Autodesk Inventor part; units mm, degrees
(part 2 of 2)
sketch "Sketch18" plane through (0, 0, -0.2) normal (0, 0, -1) x (-1, 0, 0)
  line L0 (-13.9597, 17.5749) -> (-9.7521, 15.1456) projected
  line L1 (-9.7521, 15.1456) -> (-5.5444, 17.5749) projected
  line L2 (-5.5444, 17.5749) -> (-5.5444, 22.4335) projected
  line L3 (-5.5444, 22.4335) -> (-9.7521, 24.8628) projected
  line L4 (-9.7521, 24.8628) -> (-13.9597, 22.4335) projected
  line L5 (-13.9597, 22.4335) -> (-13.9597, 17.5749) projected
  line L6 (-34.8886, 69.9757) -> (-34.8886, 76.9629) projected
  line L7 (-34.8886, 76.9629) -> (-40.9397, 80.4565) projected
  line L8 (-40.9397, 80.4565) -> (-46.9908, 76.9629) projected
  line L9 (-46.9908, 76.9629) -> (-46.9908, 69.9757) projected
  line L10 (-46.9908, 69.9757) -> (-40.9397, 66.482) projected
  line L11 (-40.9397, 66.482) -> (-34.8886, 69.9757) projected
  line L12 (-49.5403, 66.4665) -> (-49.5403, 71.3251) projected
  line L13 (-49.5403, 71.3251) -> (-53.7479, 73.7544) projected
  line L14 (-53.7479, 73.7544) -> (-57.9556, 71.3251) projected
  line L15 (-57.9556, 71.3251) -> (-57.9556, 66.4665) projected
  line L16 (-57.9556, 66.4665) -> (-53.7479, 64.0372) projected
  line L17 (-53.7479, 64.0372) -> (-49.5403, 66.4665) projected
  line L18 (0, 0) -> (-63.5, 0)
  line L19 (-63.5, 0) -> (-63.5, 88.9)
  line L20 (-63.5, 88.9) -> (0, 88.9)
  line L21 (0, 88.9) -> (0, 0)
  line L22 (-24.4329, 66.1976) -> (-24.4329, 72.4542) projected
  line L23 (-22.5603, 66.482) -> (-16.5092, 69.9757) projected
  line L24 (-16.5092, 69.9757) -> (-16.5092, 76.9629) projected
  line L25 (-16.5092, 76.9629) -> (-22.5603, 80.4565) projected
  line L26 (-22.5603, 80.4565) -> (-28.6114, 76.9629) projected
  line L27 (-28.6114, 76.9629) -> (-28.6114, 69.9757) projected
  line L28 (-28.6114, 69.9757) -> (-22.5603, 66.482) projected
  line L29 (-22.6851, 47.9436) -> (-22.6851, 40.9564) projected
  line L30 (-16.6339, 37.4628) -> (-10.5828, 40.9564) projected
  line L31 (-10.5828, 40.9564) -> (-10.5828, 47.9436) projected
  line L32 (-10.5828, 47.9436) -> (-16.6339, 51.4372) projected
  line L33 (-16.6339, 51.4372) -> (-22.6851, 47.9436) projected
  line L34 (-22.6851, 40.9564) -> (-16.6339, 37.4628) projected
  line L35 (-31.75, 54.2591) -> (-25.6989, 57.7528) projected
  line L36 (-25.6989, 57.7528) -> (-25.6989, 64.74) projected
  line L37 (-25.6989, 64.74) -> (-31.75, 68.2336) projected
  line L38 (-31.75, 68.2336) -> (-37.8011, 64.74) projected
  line L39 (-37.8011, 64.74) -> (-37.8011, 57.7528) projected
  line L40 (-37.8011, 57.7528) -> (-31.75, 54.2591) projected
  spline S0 degree 2 poles (-51.8872, 81.4609) (-51.8872, 81.2551) (-51.9037, 80.9175) (-51.9119, 80.8187) knots 0 0 0 0.5 1 1 1 projected
  spline S1 degree 2 poles (-51.9119, 80.8187) (-52.2906, 80.5635) (-53.2951, 80.2588) (-53.7315, 80.2588) knots 0 0 0 0.5 1 1 1 projected
  spline S2 degree 2 poles (-53.7315, 80.2588) (-54.1102, 80.2588) (-54.7606, 80.3988) (-55.0241, 80.6129) knots 0 0 0 0.5 1 1 1 projected
  spline S3 degree 2 poles (-55.0241, 80.6129) (-55.3864, 80.9093) (-55.7157, 81.7408) (-55.7157, 82.383) knots 0 0 0 0.5 1 1 1 projected
  spline S4 degree 2 poles (-55.7157, 82.383) (-55.7157, 83.5192) (-54.7195, 84.7213) (-53.8797, 84.7213) knots 0 0 0 0.5 1 1 1 projected
  spline S5 degree 2 poles (-53.8797, 84.7213) (-53.5174, 84.7213) (-52.8999, 84.4743) (-52.6035, 84.145) knots 0 0 0 0.5 1 1 1 projected
  spline S6 degree 2 poles (-52.6035, 84.145) (-52.2659, 83.7909) (-51.8872, 82.4901) (-51.8872, 81.4609) knots 0 0 0 0.5 1 1 1 projected
  spline S7 degree 2 poles (-56.1439, 84.8778) (-56.5885, 84.4085) (-57.0989, 83.1076) (-57.0989, 82.3254) knots 0 0 0 0.5 1 1 1 projected
  spline S8 degree 2 poles (-57.0989, 82.3254) (-57.0989, 81.428) (-56.5391, 80.1518) (-55.9957, 79.7319) knots 0 0 0 0.5 1 1 1 projected
  spline S9 degree 2 poles (-55.9957, 79.7319) (-55.5264, 79.3779) (-54.596, 79.1309) (-54.0361, 79.1309) knots 0 0 0 0.5 1 1 1 projected
  spline S10 degree 2 poles (-54.0361, 79.1309) (-53.4515, 79.1309) (-52.4635, 79.4684) (-51.9201, 79.8389) knots 0 0 0 0.5 1 1 1 projected
  spline S11 degree 2 poles (-51.9201, 79.8389) (-52.0272, 78.2087) (-53.5503, 76.4468) (-54.8841, 76.4468) knots 0 0 0 0.5 1 1 1 projected
  spline S12 degree 2 poles (-54.8841, 76.4468) (-55.2546, 76.4468) (-55.9792, 76.6197) (-56.1521, 76.7185) knots 0 0 0 0.5 1 1 1 projected
  line L41 (-56.1521, 76.7185) -> (-56.218, 76.7185) projected
  line L42 (-56.218, 76.7185) -> (-56.218, 75.4094) projected
  spline S13 degree 2 poles (-56.218, 75.4094) (-55.9545, 75.327) (-55.337, 75.2694) (-55.0653, 75.2694) knots 0 0 0 0.5 1 1 1 projected
  spline S14 degree 2 poles (-55.0653, 75.2694) (-53.8632, 75.2694) (-52.2165, 76.101) (-51.632, 76.8914) knots 0 0 0 0.5 1 1 1 projected
  spline S15 degree 2 poles (-51.632, 76.8914) (-51.0803, 77.6406) (-50.5122, 79.8966) (-50.5122, 81.1563) knots 0 0 0 0.5 1 1 1 projected
  spline S16 degree 2 poles (-50.5122, 81.1563) (-50.5122, 82.5477) (-51.0886, 84.3591) (-51.6155, 84.9189) knots 0 0 0 0.5 1 1 1 projected
  spline S17 degree 2 poles (-51.6155, 84.9189) (-52.0354, 85.3635) (-53.1716, 85.8328) (-53.8714, 85.8328) knots 0 0 0 0.5 1 1 1 projected
  spline S18 degree 2 poles (-53.8714, 85.8328) (-54.4972, 85.8328) (-55.724, 85.3306) (-56.1439, 84.8778) knots 0 0 0 0.5 1 1 1 projected
  line L43 (-52.9172, 40.9564) -> (-46.8661, 37.4628) projected
  line L44 (-46.8661, 37.4628) -> (-40.8149, 40.9564) projected
  line L45 (-40.8149, 40.9564) -> (-40.8149, 47.9436) projected
  line L46 (-40.8149, 47.9436) -> (-46.8661, 51.4372) projected
  line L47 (-46.8661, 51.4372) -> (-52.9172, 47.9436) projected
  line L48 (-52.9172, 47.9436) -> (-52.9172, 40.9564) projected
  line L49 (-37.8011, 47.9436) -> (-37.8011, 40.9564) projected
  line L50 (-37.8011, 40.9564) -> (-31.75, 37.4628) projected
  line L51 (-31.75, 37.4628) -> (-25.6989, 40.9564) projected
  line L52 (-25.6989, 40.9564) -> (-25.6989, 47.9436) projected
  line L53 (-25.6989, 47.9436) -> (-31.75, 51.4372) projected
  line L54 (-31.75, 51.4372) -> (-37.8011, 47.9436) projected
  line L55 (-31.75, 34.6409) -> (-37.8011, 31.1472) projected
  line L56 (-37.8011, 31.1472) -> (-37.8011, 24.16) projected
  line L57 (-37.8011, 24.16) -> (-31.75, 20.6664) projected
  line L58 (-31.75, 20.6664) -> (-25.6989, 24.16) projected
  line L59 (-25.6989, 24.16) -> (-25.6989, 31.1472) projected
  line L60 (-25.6989, 31.1472) -> (-31.75, 34.6409) projected
  line L61 (-34.8886, 11.9371) -> (-34.8886, 18.9243) projected
  line L62 (-34.8886, 18.9243) -> (-40.9397, 22.418) projected
  line L63 (-40.9397, 22.418) -> (-46.9908, 18.9243) projected
  line L64 (-46.9908, 18.9243) -> (-46.9908, 11.9371) projected
  line L65 (-46.9908, 11.9371) -> (-40.9397, 8.4435) projected
  line L66 (-40.9397, 8.4435) -> (-34.8886, 11.9371) projected
  line L67 (-28.6114, 11.9371) -> (-22.5603, 8.4435) projected
  line L68 (-22.5603, 8.4435) -> (-16.5092, 11.9371) projected
  line L69 (-16.5092, 11.9371) -> (-16.5092, 18.9243) projected
  line L70 (-16.5092, 18.9243) -> (-22.5603, 22.418) projected
  line L71 (-22.5603, 22.418) -> (-28.6114, 18.9243) projected
  line L72 (-28.6114, 18.9243) -> (-28.6114, 11.9371) projected
  spline S19 degree 2 poles (-11.6128, 7.7837) (-11.6128, 7.9895) (-11.5963, 8.3271) (-11.5881, 8.4259) knots 0 0 0 0.5 1 1 1 projected
  spline S20 degree 2 poles (-11.5881, 8.4259) (-11.2094, 8.6811) (-10.2049, 8.9857) (-9.7685, 8.9857) knots 0 0 0 0.5 1 1 1 projected
  spline S21 degree 2 poles (-9.7685, 8.9857) (-9.3898, 8.9857) (-8.7394, 8.8458) (-8.4759, 8.6317) knots 0 0 0 0.5 1 1 1 projected
  spline S22 degree 2 poles (-8.4759, 8.6317) (-8.1136, 8.3353) (-7.7843, 7.5037) (-7.7843, 6.8615) knots 0 0 0 0.5 1 1 1 projected
  spline S23 degree 2 poles (-7.7843, 6.8615) (-7.7843, 5.7253) (-8.7805, 4.5233) (-9.6203, 4.5233) knots 0 0 0 0.5 1 1 1 projected
  spline S24 degree 2 poles (-9.6203, 4.5233) (-9.9826, 4.5233) (-10.6001, 4.7703) (-10.8965, 5.0996) knots 0 0 0 0.5 1 1 1 projected
  spline S25 degree 2 poles (-10.8965, 5.0996) (-11.2341, 5.4536) (-11.6128, 6.7545) (-11.6128, 7.7837) knots 0 0 0 0.5 1 1 1 projected
  spline S26 degree 2 poles (-7.3561, 4.3668) (-6.9115, 4.8361) (-6.4011, 6.137) (-6.4011, 6.9192) knots 0 0 0 0.5 1 1 1 projected
  spline S27 degree 2 poles (-6.4011, 6.9192) (-6.4011, 7.8166) (-6.9609, 9.0928) (-7.5043, 9.5127) knots 0 0 0 0.5 1 1 1 projected
  spline S28 degree 2 poles (-7.5043, 9.5127) (-7.9736, 9.8667) (-8.904, 10.1137) (-9.4639, 10.1137) knots 0 0 0 0.5 1 1 1 projected
  spline S29 degree 2 poles (-9.4639, 10.1137) (-10.0485, 10.1137) (-11.0365, 9.7762) (-11.5799, 9.4057) knots 0 0 0 0.5 1 1 1 projected
  spline S30 degree 2 poles (-11.5799, 9.4057) (-11.4728, 11.0359) (-9.9497, 12.7978) (-8.6159, 12.7978) knots 0 0 0 0.5 1 1 1 projected
  spline S31 degree 2 poles (-8.6159, 12.7978) (-8.2454, 12.7978) (-7.5208, 12.6249) (-7.3479, 12.5261) knots 0 0 0 0.5 1 1 1 projected
  line L73 (-7.3479, 12.5261) -> (-7.282, 12.5261) projected
  line L74 (-7.282, 12.5261) -> (-7.282, 13.8352) projected
  spline S32 degree 2 poles (-7.282, 13.8352) (-7.5455, 13.9175) (-8.163, 13.9752) (-8.4347, 13.9752) knots 0 0 0 0.5 1 1 1 projected
  spline S33 degree 2 poles (-8.4347, 13.9752) (-9.6368, 13.9752) (-11.2835, 13.1436) (-11.868, 12.3532) knots 0 0 0 0.5 1 1 1 projected
  spline S34 degree 2 poles (-11.868, 12.3532) (-12.4197, 11.604) (-12.9878, 9.348) (-12.9878, 8.0883) knots 0 0 0 0.5 1 1 1 projected
  spline S35 degree 2 poles (-12.9878, 8.0883) (-12.9878, 6.6969) (-12.4114, 4.8855) (-11.8845, 4.3257) knots 0 0 0 0.5 1 1 1 projected
  spline S36 degree 2 poles (-11.8845, 4.3257) (-11.4646, 3.881) (-10.3284, 3.4117) (-9.6286, 3.4117) knots 0 0 0 0.5 1 1 1 projected
  spline S37 degree 2 poles (-9.6286, 3.4117) (-9.0028, 3.4117) (-7.776, 3.914) (-7.3561, 4.3668) knots 0 0 0 0.5 1 1 1 projected
  constraints: 8 end point, 2 parallel, 1 horizontal, 1 perpendicular, 38 other
extrude "Extrusion21" add sketch "Sketch18" along normal blind 0.4 bodies 3
fillet "Fillet2" radius 3.175 8 edges at (63.5, 0, 0.2) (63.5, 88.9, 0.2) (0, 0, 0.2) (0, 88.9, 0.2) (63.5, 0, -0.3) (63.5, 88.9, -0.3) (0, 0, -0.3) (0, 88.9, -0.3)
